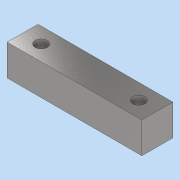
# Autodesk Inventor part: LoadCell
Saved by Autodesk Inventor 2021 (Build 250183000, 183)
## iProperties
Created: 2021-02-01
Part Number: LoadCell
Material: Generic
Document SubType Name: Modeling
Designer: garre
Density: 1 g/cm^3
Appearance: Default
Author: garre
Autodesk Inventor part; units mm, degrees
ref_plane "YZ Plane" through (0, 0, 0) normal (1, 0, 0) x (0, 1, 0)
ref_plane "XZ Plane" through (0, 0, 0) normal (0, 1, 0) x (-1, 0, 0)
ref_plane "XY Plane" through (0, 0, 0) normal (0, 0, 1) x (1, 0, 0)
sketch "Sketch1" plane through (0, 0, 0) normal (0, 0, 1) x (1, 0, 0)
  line L0 (0, 0) -> (55.245, 0)
  line L1 (55.245, 0) -> (55.245, 12.7)
  line L2 (55.245, 12.7) -> (0, 12.7)
  line L3 (0, 12.7) -> (0, 0)
  dimension "d0" = 12.7
  dimension "d1" = 55.245
  constraints: 8 end point, 2 parallel, 1 horizontal, 1 perpendicular
  measures "d0" distance of L2.end L0.start
  measures "d1" distance of L1.end L2.end
extrude "Extrusion1" add sketch "Sketch1" against normal blind 12.7
sketch "Sketch2" plane through (0, 12.7, 0) normal (0, 1, 0) x (1, 0, 0)
  line L0 (0, 0) -> (0, 12.7) projected
  line L1 (0, 6.35) -> (57.5321, 6.35)
  circle A0 centre (7.62, 6.35) radius 2.5
  circle A1 centre (47.625, 6.35) radius 2.5
  dimension "d4" = 40.005
  dimension "d5" = 5
  dimension "d6" = 5
  dimension "d7" = 7.62
  constraints: 2 centre point, 2 end point, 2 point on line, 1 horizontal, 1 midpoint
  measures "d4" distance of A1.centre A0.centre
  measures "d5" diameter of A0
  measures "d6" diameter of A1
  measures "d7" distance from line of L0 A0.centre
extrude "Extrusion2" cut sketch "Sketch2" against normal up to surface (12.7 mm away)
equation "\"d0\" = loadCellWidth"
equation "\"d2\" = loadCellWidth"
equation "\"loadCellWidth\" = 12.7"
body "Solid1"
